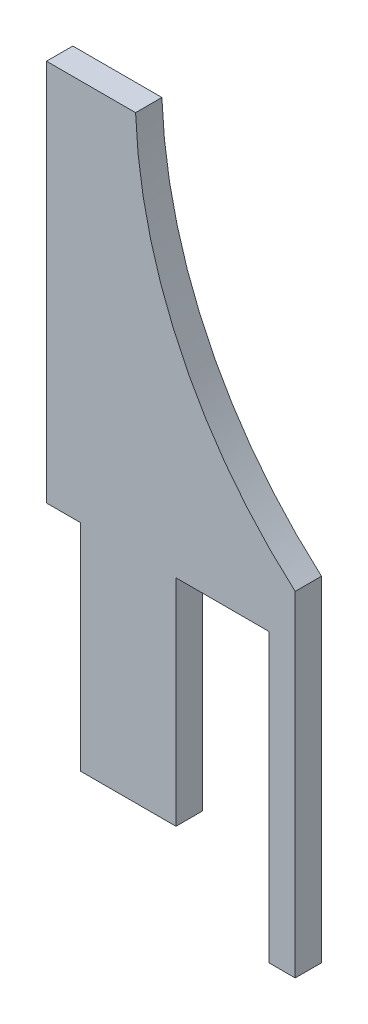
# Autodesk Inventor part: brazos
Saved by Autodesk Inventor 2015 (Build 190159000, 159)
## iProperties
Created: 2017-10-02
Part Number: brazos
Material: Generic
Document SubType Name: Modeling
Designer: macbook
Density: 1 g/cm^3
Appearance: Default
Author: macbook
Autodesk Inventor part; units mm, degrees
ref_plane "YZ Plane" through (0, 0, 0) normal (1, 0, 0) x (0, 1, 0)
ref_plane "XZ Plane" through (0, 0, 0) normal (0, 1, 0) x (-1, 0, 0)
ref_plane "XY Plane" through (0, 0, 0) normal (0, 0, 1) x (1, 0, 0)
sketch "Sketch1" plane through (0, 0, 0) normal (0, 0, 1) x (1, 0, 0)
  arc A0 (18.6268, 80) -> (52, 10) centre (115.8042, 83.3748) ccw
  line L0 (0, 80) -> (18.6268, 80)
  line L1 (46.5, 0) -> (27.071, 0)
  line L2 (7.071, 0) -> (0, 0)
  line L3 (7.071, 0) -> (7.071, -45)
  line L4 (7.071, -45) -> (27.071, -45)
  line L5 (27.071, -45) -> (27.071, 0)
  line L6 (46.5, 0) -> (46.5, -60)
  line L7 (46.5, -60) -> (52, -60)
  line L8 (52, -60) -> (52, 0)
  line L9 (0, 80) -> (0, 0)
  line L10 (52, 10) -> (52, 0)
  dimension "d22" = 52
  dimension "d23" = 19.429
  dimension "d24" = 45
  dimension "d25" = 60
  constraints: 22 end point, 4 perpendicular, 3 horizontal, 3 vertical, 2 point on circle, 1 centre point, 1 parallel, 1 point on line
  measures "d22" distance of L2.end L8.end
  measures "d23" distance of L1.start L1.end
  measures "d24" distance of L3.start L3.end
  measures "d25" distance of L1.start L6.end
extrude "Extrusion2" add sketch "Sketch1" along normal blind 5.5
body "Solid2"
